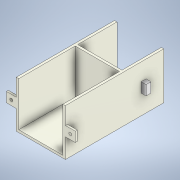
# Autodesk Inventor part: Torre Motor
Saved by Autodesk Inventor 2021 (Build 250183000, 183)
## iProperties
Created: 2021-02-25
Part Number: Torre Motor
Material: Plástico ABS
Document SubType Name: Modeling
Designer: Marc
Density: 1.06 g/cm^3
Appearance: Suave - Blanco
Author: Marc
Autodesk Inventor part; units mm, degrees
ref_plane "YZ Plane" through (0, 0, 0) normal (1, 0, 0) x (0, 1, 0)
ref_plane "XZ Plane" through (0, 0, 0) normal (0, 1, 0) x (-1, 0, 0)
ref_plane "XY Plane" through (0, 0, 0) normal (0, 0, 1) x (1, 0, 0)
sketch "Boceto1" plane through (0, 0, 0) normal (0, 0, 1) x (1, 0, 0)
  line L0 (-22.5, 22.5) -> (-22.5, -22.5)
  line L1 (-22.5, -22.5) -> (22.5, -22.5)
  line L2 (22.5, -22.5) -> (22.5, 22.5)
  line L3 (-25, 22.5) -> (-25, -25)
  line L4 (-25, -25) -> (25, -25)
  line L5 (25, -25) -> (25, 22.5)
  line L6 (22.5, 22.5) -> (25, 22.5)
  line L7 (-22.5, 22.5) -> (-25, 22.5)
  constraints: 16 end point, 2 parallel, 1 perpendicular, 1 point on line
extrude "Extrusión1" add sketch "Boceto1" along normal blind 100
sketch "Boceto2" plane through (-22.5, -22.5, 0) normal (0, 1, 0) x (1, 0, 0)
  line L0 (-2.5, -100) -> (47.5, -100) projected
  line L1 (22.5, -40) -> (45, -40)
  line L2 (45, 0) -> (45, -100) projected
  line L3 (0, 0) -> (0, -100) projected
  line L4 (0, -40) -> (22.5, -40)
  line L5 (22.5, -42.5) -> (45, -42.5)
  line L6 (22.5, -42.5) -> (0, -42.5)
  line L7 (45, -40) -> (45, -42.5)
  line L8 (0, -40) -> (0, -42.5)
  point P0 (22.5, 0)
  dimension "d10" = 2.5
  constraints: 12 end point, 6 point on line, 3 perpendicular, 1 parallel
  measures "d10" distance of L1.start L5.start
extrude "Extrusión2" add sketch "Boceto2" along normal blind 45 contours L3 L4 L1 L2 L5 L6
sketch "Boceto3" plane through (25, -25, 0) normal (1, 0, 0) x (0, 0, -1)
  line L0 (-100, 2.5) -> (-100, 47.5) projected
  line L1 (-100, 25) -> (-100, 20)
  line L2 (-100, 25) -> (-100, 30)
  line L3 (-100, 30) -> (-98, 30)
  line L4 (-98, 30) -> (-98, 20)
  line L5 (-98, 20) -> (-100, 20)
  point P0 (0, 25)
  dimension "d13" = 5
  dimension "d14" = 5
  dimension "d15" = 2
  constraints: 10 end point, 3 perpendicular, 2 point on line, 1 midpoint
  measures "d13" distance of L1.start L1.end
  measures "d14" distance of L1.start L2.end
  measures "d15" distance of L2.end L3.end
sketch "Boceto4" plane through (-25, -25, 0) normal (-1, 0, 0) x (0, 0, 1)
  line L0 (100, 2.5) -> (100, 47.5) projected
  line L1 (100, 25) -> (100, 20)
  line L2 (100, 25) -> (100, 30)
  line L3 (100, 30) -> (98, 30)
  line L4 (98, 30) -> (98, 20)
  line L5 (98, 20) -> (100, 20)
  point P0 (0, 25)
  dimension "d16" = 5
  dimension "d17" = 5
  dimension "d18" = 2
  constraints: 10 end point, 3 perpendicular, 2 point on line, 1 midpoint
  measures "d16" distance of L1.start L1.end
  measures "d17" distance of L1.start L2.end
  measures "d18" distance of L2.end L3.end
extrude "Extrusión3" add sketch "Boceto4" along normal blind 10
extrude "Extrusión4" add sketch "Boceto3" along normal blind 10
sketch "Boceto5" plane through (25, -5, 98) normal (0, 0, -1) x (-1, 0, 0)
  line L0 (0, 0) -> (-10, 0) projected
  line L1 (0, 10) -> (0, 27.5) projected
  line L2 (0, 10) -> (-10, 10)
  line L3 (50, 0) -> (50, -20) projected
  line L4 (50, 0) -> (59.9457, 0)
  line L5 (50, 27.5) -> (50, 10) projected
  circle A0 centre (-5, 5) radius 1.5
  circle A1 centre (54.9729, 5) radius 1.5
  point P0 (25, 5)
  dimension "d23" = 3
  dimension "d24" = 3
  constraints: 4 end point, 2 centre point, 2 perpendicular
  measures "d23" diameter of A0
  measures "d24" diameter of A1
extrude "Extrusión5" cut sketch "Boceto5" against normal through all
sketch "Boceto7" plane through (25, -25, 0) normal (1, 0, 0) x (0, 0, -1)
  line L0 (-17.98, 25) -> (-17.98, 30)
  line L1 (-17.98, 30) -> (-17.98, 25)
  line L2 (-17.98, 25) -> (-17.98, 20)
  line L3 (-17.98, 20) -> (-22.98, 20)
  line L4 (-22.98, 20) -> (-22.98, 30)
  line L5 (-22.98, 30) -> (-17.98, 30)
  point P0 (0, 25)
  dimension "d27" = 17.98
  dimension "d28" = 5
  dimension "d29" = 5
  dimension "d30" = 5
  constraints: 12 end point, 3 perpendicular, 1 collinear, 1 point on line, 1 vertical
  measures "d27" distance of point (0, 25) L0.start
  measures "d28" distance of L0.start L0.end
  measures "d29" distance of L0.start L2.end
  measures "d30" distance of L2.end L3.end
sketch "Boceto8" plane through (-25, -25, 0) normal (-1, 0, 0) x (0, 0, 1)
  line L0 (0, 25) -> (17.98, 25)
  line L1 (17.98, 25) -> (17.98, 20)
  line L2 (17.98, 20) -> (22.98, 20)
  line L3 (22.98, 20) -> (22.98, 30)
  line L4 (22.98, 30) -> (17.98, 30)
  line L5 (17.98, 30) -> (17.98, 25)
  dimension "d31" = 17.98
  dimension "d32" = 5
  dimension "d33" = 5
  dimension "d34" = 10
  dimension "d35" = 5
  dimension "d36" = 5
  constraints: 12 end point, 3 perpendicular, 1 horizontal, 1 point on line
  measures "d31" distance of L0.start L0.end
  measures "d32" distance of L0.end L1.end
  measures "d33" distance of L1.end L2.end
  measures "d34" distance of L2.end L3.end
  measures "d35" distance of L3.end L4.end
  measures "d36" distance of L4.end L0.end
extrude "Extrusión6" add sketch "Boceto8" along normal blind 5
extrude "Extrusión7" add sketch "Boceto7" along normal blind 5
